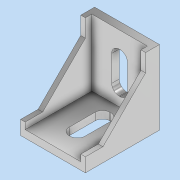
# Autodesk Inventor part: KE HOC NHOM DINH HINH
Saved by Autodesk Inventor 2021 (Build 250183000, 183)
## iProperties
Created: 2021-04-01
Part Number: KE HOC NHOM DINH HINH
Material: Generic
Document SubType Name: Modeling
Designer: 41601100
Density: 1 g/cm^3
Appearance: Default
Author: 41601100
Autodesk Inventor part; units mm, degrees
ref_plane "YZ Plane" through (0, 0, 0) normal (1, 0, 0) x (0, 1, 0)
ref_plane "XZ Plane" through (0, 0, 0) normal (0, 1, 0) x (-1, 0, 0)
ref_plane "XY Plane" through (0, 0, 0) normal (0, 0, 1) x (1, 0, 0)
sketch "Sketch1" plane through (0, 0, 0) normal (0, 1, 0) x (-1, 0, 0)
  line L0 (0, 0) -> (17.5, 0)
  line L1 (17.5, 0) -> (17.5, -20)
  line L2 (17.5, -20) -> (-17.5, -20)
  line L3 (-17.5, -20) -> (-17.5, 20)
  line L4 (-17.5, 20) -> (17.5, 20)
  line L5 (17.5, 20) -> (17.5, 0)
  line L6 (15, -17.5) -> (15, 0)
  line L7 (15, 0) -> (15, 17.5)
  line L8 (15, 17.5) -> (-15, 17.5)
  line L9 (-15, 17.5) -> (-15, -17.5)
  line L10 (-15, -17.5) -> (15, -17.5)
  line L11 (0, 0) -> (0, 11)
  line L12 (0, 0) -> (0, -11)
  line L13 (0, 0) -> (4.25, 0)
  line L14 (4.25, 0) -> (4.25, -7)
  line L15 (0.25, -11) -> (-0.25, -11)
  line L16 (-4.25, -7) -> (-4.25, 7)
  line L17 (-0.25, 11) -> (0.25, 11)
  line L18 (4.25, 7) -> (4.25, 0)
  arc A0 (4.25, 7) -> (0.25, 11) centre (0.25, 7) ccw
  arc A1 (-0.25, 11) -> (-4.25, 7) centre (-0.25, 7) ccw
  arc A2 (0.25, -11) -> (4.25, -7) centre (0.25, -7) ccw
  arc A3 (-4.25, -7) -> (-0.25, -11) centre (-0.25, -7) ccw
  point P0 (4.25, -11)
  point P1 (-4.25, -11)
  point P2 (4.25, 11)
  dimension "d2" = 17.5
  dimension "d3" = 20
  dimension "d4" = 35
  dimension "d5" = 40
  dimension "d6" = 35
  dimension "d7" = 2.5
  dimension "d8" = 11
  dimension "d9" = 11
  dimension "d10" = 4.25
  dimension "d11" = 8.5
  dimension "d12" = 4
  constraints: 38 end point, 9 perpendicular, 9 point on line, 8 point on circle, 8 tangent, 4 centre point, 3 equal radius, 3 vertical, 2 collinear, 1 horizontal, 4 other
  measures "d2" distance of L0.start L0.end
  measures "d3" distance of L0.end L1.end
  measures "d4" distance of L1.end L2.end
  measures "d5" distance of L2.end L3.end
  measures "d6" distance of L3.end L4.end
  measures "d7" distance between parallel lines of L1 L6
  measures "d8" distance of L0.start L11.end
  measures "d9" distance of L0.start L12.end
  measures "d10" distance of L0.start L13.end
  measures "d11" distance of point (4.25, -11) point (-4.25, -11)
  measures "d12" radius of A0
extrude "Extrusion1" add sketch "Sketch1" along normal blind 4 contours L6 L10 L9 L8 L7 | L1 L2 L3 L4 L5
sketch "Sketch2" plane through (0, 4, 0) normal (0, 1, 0) x (1, 0, 0)
  line L0 (-17.5, -20) -> (17.5, -20) projected
  line L1 (17.5, -20) -> (17.5, 20) projected
  line L2 (17.5, 20) -> (-17.5, 20) projected
  line L3 (-17.5, 20) -> (-17.5, -20) projected
  line L4 (-4.25, -7) -> (-4.25, 7) projected
  arc A0 (-0.25, 11) -> (-4.25, 7) centre (-0.25, 7) ccw projected
  line L5 (-0.25, 11) -> (0.25, 11) projected
  arc A1 (4.25, 7) -> (0.25, 11) centre (0.25, 7) ccw projected
  line L6 (4.25, 7) -> (4.25, -7) projected
  arc A2 (0.25, -11) -> (4.25, -7) centre (0.25, -7) ccw projected
  line L7 (0.25, -11) -> (-0.25, -11) projected
  arc A3 (-4.25, -7) -> (-0.25, -11) centre (-0.25, -7) ccw projected
  line L8 (-17.5, 20) -> (-17.5, -20) projected
  line L9 (-17.5, 20) -> (-17.5, 16)
  line L10 (-17.5, 16) -> (17.5, 16)
  line L11 (17.5, -20) -> (17.5, 20) projected
  point P0 (0, 0)
  dimension "d15" = 4
  constraints: 4 end point, 2 point on line, 1 perpendicular
  measures "d15" distance of L2.end L9.end
extrude "Extrusion2" add sketch "Sketch2" along normal blind 36 contours L3 L2 L1 L10
sketch "Sketch3" plane through (17.5, 0, -20) normal (0, 0, -1) x (-1, 0, 0)
  line L0 (0, 0) -> (35, 0) projected
  line L1 (35, 0) -> (35, 40) projected
  line L2 (0, 40) -> (35, 40) projected
  line L3 (0, 0) -> (0, 40) projected
  line L4 (17.5, 0) -> (17.5, 40)
  line L5 (35, 40) -> (0, 40) projected
  line L6 (17.5, 20) -> (17.5, 9)
  line L7 (17.5, 20) -> (17.5, 31)
  line L8 (17.5, 31) -> (17.25, 31)
  line L9 (13.25, 27) -> (13.25, 13)
  line L10 (17.25, 9) -> (17.75, 9)
  line L11 (21.75, 13) -> (21.75, 27)
  line L12 (17.75, 31) -> (17.5, 31)
  arc A0 (13.25, 13) -> (17.25, 9) centre (17.25, 13) ccw
  arc A1 (17.75, 9) -> (21.75, 13) centre (17.75, 13) ccw
  arc A2 (17.25, 31) -> (13.25, 27) centre (17.25, 27) ccw
  arc A3 (21.75, 27) -> (17.75, 31) centre (17.75, 27) ccw
  point P0 (13.25, 31)
  point P1 (13.25, 9)
  point P2 (21.75, 9)
  point P3 (21.75, 31)
  dimension "d18" = 11
  dimension "d19" = 11
  dimension "d20" = 4.25
  dimension "d21" = 22
  dimension "d22" = 8.5
  dimension "d23" = 4
  constraints: 16 end point, 11 point on line, 8 point on circle, 8 tangent, 5 perpendicular, 4 centre point, 3 equal radius, 2 midpoint
  measures "d18" distance of L6.start L6.end
  measures "d19" distance of L6.start L7.end
  measures "d20" distance of L7.end point (13.25, 31)
  measures "d21" distance of point (13.25, 31) point (13.25, 9)
  measures "d22" distance of point (13.25, 9) point (21.75, 9)
  measures "d23" radius of A0
extrude "Extrusion3" cut sketch "Sketch3" against normal blind 4 contours L10 A0 L9 A2 L8 L4 | L4 L12 A3 L11 A1 L10
sketch "Sketch4" plane through (17.5, 0, 20) normal (1, 0, 0) x (0, 0, -1)
  line L0 (0, 0) -> (40, 0) projected
  line L1 (40, 0) -> (40, 40) projected
  line L2 (36, 40) -> (40, 40) projected
  line L3 (36, 4) -> (36, 40) projected
  line L4 (0, 4) -> (36, 4) projected
  line L5 (0, 0) -> (0, 4) projected
  line L6 (36, 4) -> (0, 4) projected
  line L7 (0, 4) -> (0, 7.5)
  line L8 (0, 7.5) -> (9.5, 7.5)
  line L9 (36, 4) -> (36, 40) projected
  line L10 (36, 40) -> (32.5, 40)
  line L11 (32.5, 40) -> (32.5, 30.5)
  line L12 (0, 7.5) -> (9.5, 7.5)
  line L13 (32.5, 40) -> (32.5, 30.5)
  line L14 (32.5, 30.5) -> (9.5, 7.5)
  point P0 (20, 0)
  dimension "d26" = 3.5
  dimension "d27" = 3.5
  dimension "d28" = 9.5
  dimension "d29" = 9.5
  constraints: 14 end point, 2 perpendicular, 1 horizontal, 1 vertical
  measures "d26" distance of L4.start L7.end
  measures "d27" distance of L2.start L10.end
  measures "d28" distance of L8.end L7.end
  measures "d29" distance of L11.end L10.end
extrude "Extrusion4" add sketch "Sketch4" against normal blind 2.5 contours L7 L8 L14 L11 L10 L3 L4
mirror "Mirror1" about plane through (0, 0, 0) normal (1, 0, 0) of "Extrusion4"
ref_plane "Work Plane1" through (0, 0, 0) normal (1, 0, 0) x (0, 1, 0)
body "Solid1"
